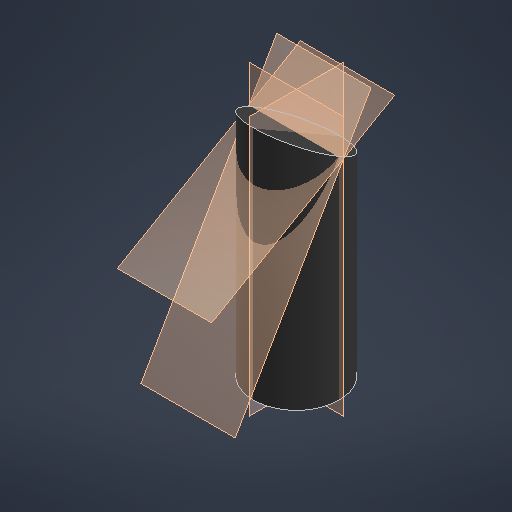
# Autodesk Inventor part: Camera encasing
Saved by Autodesk Inventor 2026.2 (Build 302298010, 298A)
## iProperties
Created: 2026-04-01
Part Number: Camera encasing
Material: Rubber
Document SubType Name: Modeling
Designer: piete
Density: 0.93 g/cm^3
Appearance: Rubber - Black
Author: piete
Autodesk Inventor part; units mm, degrees
ref_plane "XZ Plane" through (0, 0, 0) normal (0, 1, 0) x (-1, 0, 0)
sketch "Sketch1" plane through (0, 0, 0) normal (0, 1, 0) x (-1, 0, 0)
  circle A0 centre (0, 0) radius 4
  dimension "d0" = 8
  constraints: 1 centre point, 1 coincident
  measures "d0" diameter of A0
extrude "Extrusion1" add sketch "Sketch1" along normal blind 20
sketch "Sketch2" plane through (0, 20, 0) normal (0, 1, 0) x (1, 0, 0)
  circle A0 centre (0, 0) radius 4
  dimension "d3" = 8
  constraints: 1 centre point, 1 coincident
  measures "d3" diameter of A0
extrude "Extrusion2" add sketch "Sketch2" along normal blind 2
sketch "Sketch3" plane through (0, 0, 0) normal (1, 0, 0) x (0, 1, 0)
  line L0 (22, -4) -> (22, 4) projected
  line L1 (22, 4) -> (17.3812, -4)
  line L2 (0, -4) -> (22, -4) projected
  line L3 (22, 4) -> (31.2376, 4) construction
  line L4 (17.3812, -4) -> (22, -4)
  line L5 (22, 4) -> (22, -4)
  point P0 (0, 0)
  dimension "d6" = 120
  constraints: 8 end point, 2 point on line, 1 equal length, 1 horizontal, 1 perpendicular
  measures "d6" angle of L1 L3
extrude "Extrusion3" cut sketch "Sketch3" along normal through all both and the other way through all
sketch "Sketch4" plane through (0, 0, 0) normal (1, 0, 0) x (0, 1, 0)
  point P0 (0, 0)
ref_plane "Work Plane2" through (0, 19.6906, 0) normal (0, 0.5, 0.8660254) x (-1, 0, 0)
ref_plane "Work Plane1" through (0, 19.6906, 0) normal (0, 0.8660254, 0.5) x (1, 0, 0)
body "Solid1"
